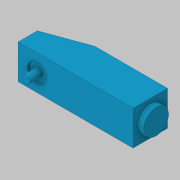
# Autodesk Inventor part: B7-A3
Saved by Autodesk Inventor 2018.1 (Build 221171000, 171)
## iProperties
Created: 2018-06-23
Part Number: B7-A3
Material: Všeobecné
Document SubType Name: Modeling
Designer: PS
Density: 1 g/cm^3
Appearance: Výchozí
Author: PS
Autodesk Inventor part; units mm, degrees
ref_plane "YZ Plane" through (0, 0, 0) normal (1, 0, 0) x (0, 1, 0)
ref_plane "XZ Plane" through (0, 0, 0) normal (0, 1, 0) x (-1, 0, 0)
ref_plane "XY Plane" through (0, 0, 0) normal (0, 0, 1) x (1, 0, 0)
sketch "Náčrt1" plane through (0, 0, 0) normal (0, 0, 1) x (1, 0, 0)
  line L0 (0, 0) -> (600, 0)
  line L1 (600, 0) -> (600, -180)
  line L2 (600, -180) -> (0, -180)
  line L3 (0, -180) -> (0, 0)
  line L4 (0, -80) -> (220, 0)
  dimension "d43" = 600
  dimension "d44" = 180
  dimension "d45" = 100
  dimension "d46" = 220
  constraints: 10 end point, 2 parallel, 2 point on line, 1 horizontal, 1 perpendicular
  measures "d43" distance of L1.end L2.end
  measures "d44" distance of L0.end L1.end
  measures "d45" distance from line of L4.start L2
  measures "d46" distance from line of L4.end L3
extrude "Vysunutí1" add sketch "Náčrt1" against normal blind 180 contours L0 L1 L2 L3 L4
sketch "Náčrt6" plane through (600, -180, 0) normal (1, 0, 0) x (0, 0, -1)
  line L0 (180, 180) -> (180, 0) projected
  line L1 (0, 0) -> (0, 180) projected
  line L2 (180, 180) -> (0, 0) construction
  circle A0 centre (90, 90) radius 65
  dimension "d47" = 130
  constraints: 2 end point, 1 centre point, 1 midpoint
  measures "d47" diameter of A0
extrude "Vysunutí6" add sketch "Náčrt6" along normal blind 30
sketch "Náčrt7" plane through (0, -180, 0) normal (0, -1, 0) x (1, 0, 0)
  circle A0 centre (100, -90) radius 50
  line L0 (0, 0) -> (0, -180) projected
  line L1 (0, -90) -> (285.9708, -90) construction
  dimension "d50" = 100
  dimension "d51" = 100
  constraints: 2 end point, 1 centre point, 1 horizontal, 1 midpoint
  measures "d50" diameter of A0
  measures "d51" distance from line of A0.centre L0
extrude "Vysunutí7" cut sketch "Náčrt7" against normal blind 10
sketch "Náčrt8" plane through (100, -170, -90) normal (0, -1, 0) x (1, 0, 0)
  circle A0 centre (0, 0) radius 20
  point P0 (-100, 90)
  dimension "d54" = 40
  constraints: 1 centre point
  measures "d54" diameter of A0
extrude "Vysunutí8" add sketch "Náčrt8" along normal blind 70
sketch "Náčrt5" plane through (0, 0, 0) normal (0, 0, 1) x (-1, 0, 0)
  circle A0 centre (0, 0) radius 65
  dimension "d40" = 130
  constraints: 1 centre point, 1 coincident
  measures "d40" diameter of A0
